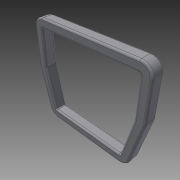
# Autodesk Inventor part: y_carryage_nut_holder_a_zip_tie
Saved by Autodesk Inventor 2014 (Build 180170000, 170)
## iProperties
Created: 2014-01-11
Part Number: y_carryage_nut_holder_a_zip_tie
Material: Generic
Document SubType Name: Modeling
Designer: buben
Density: 1 g/cm^3
Appearance: Default
Author: buben
Autodesk Inventor part; units mm, degrees
ref_plane "YZ Plane" through (0, 0, 0) normal (1, 0, 0) x (0, 1, 0)
ref_plane "XZ Plane" through (0, 0, 0) normal (0, 1, 0) x (-1, 0, 0)
ref_plane "XY Plane" through (0, 0, 0) normal (0, 0, 1) x (1, 0, 0)
sketch "Sketch1" plane through (0, 0, 0) normal (0, 1, 0) x (-1, 0, 0)
  line L0 (-7.8, 0) -> (7.8, 0)
  arc A0 (8, -0.2) -> (7.8, 0) centre (7.8, -0.2) ccw
  arc A1 (-7.8, 0) -> (-8, -0.2) centre (-7.8, -0.2) ccw
  line L1 (-8, -0.2) -> (-8, -6)
  line L2 (8, -0.2) -> (8, -6)
  arc A2 (-8, -6) -> (-7.9953, -6.043) centre (-7.8, -6) ccw
  arc A3 (7.9953, -6.043) -> (8, -6) centre (7.8, -6) ccw
  line L3 (-7.9953, -6.043) -> (-6.5, -12.843)
  line L4 (7.9953, -6.043) -> (6.5, -12.843)
  arc A4 (-6.5, -12.843) -> (-6.3047, -13) centre (-6.3047, -12.8) ccw
  line L5 (-6.3047, -13) -> (6.3047, -13)
  arc A5 (6.3047, -13) -> (6.5, -12.843) centre (6.3047, -12.8) ccw
  line L6 (-9.5, -6) -> (-9.5, -0.2)
  arc A6 (-7.8, 1.5) -> (-9.5, -0.2) centre (-7.8, -0.2) ccw
  line L7 (-7.8, 1.5) -> (7.8, 1.5)
  arc A7 (9.5, -0.2) -> (7.8, 1.5) centre (7.8, -0.2) ccw
  line L8 (9.5, -0.2) -> (9.5, -6)
  arc A8 (9.4603, -6.3651) -> (9.5, -6) centre (7.8, -6) ccw
  line L9 (9.4603, -6.3651) -> (7.965, -13.1651)
  arc A9 (6.3047, -14.5) -> (7.965, -13.1651) centre (6.3047, -12.8) ccw
  line L10 (6.3047, -14.5) -> (-6.3047, -14.5)
  arc A10 (-7.965, -13.1651) -> (-6.3047, -14.5) centre (-6.3047, -12.8) ccw
  line L11 (-7.965, -13.1651) -> (-9.4603, -6.3651)
  arc A11 (-9.5, -6) -> (-9.4603, -6.3651) centre (-7.8, -6) ccw
  point P0 (0, 0)
  point P1 (0, 0)
  point P2 (0, -13)
  dimension "d0" = 0.2
  dimension "d1" = 0.2
  dimension "d2" = 16
  dimension "d3" = 6
  dimension "d4" = 0.2
  dimension "d5" = 0.2
  dimension "d6" = 0.2
  dimension "d7" = 0.2
  dimension "d8" = 13
  dimension "d9" = 13
  dimension "d10" = 1.5
  constraints: 24 end point, 24 point on circle, 12 centre point, 12 tangent, 4 parallel, 2 midpoint, 2 perpendicular, 1 coincident, 1 horizontal, 1 horizontal alignment, 1 vertical alignment, 11 other
  measures "d0" radius of A1
  measures "d1" radius of A0
  measures "d2" distance of L2.start L1.start
  measures "d3" vertical distance of L1.end L0.start
  measures "d4" radius of A2
  measures "d5" radius of A4
  measures "d6" radius of A5
  measures "d7" radius of A3
  measures "d8" distance between parallel lines of L5 L0
  measures "d9" distance of L4.end L3.end
  measures "d10" distance between parallel lines of L1 L6
extrude "Extrusion1" add sketch "Sketch1" along normal blind 2
fillet "Fillet1" radius 0.3 48 edges at (9.0021, 2, 1.0021) (9.5, 2, -3.1) (9.4901, 2, -6.1836) (8.7127, 2, -9.7651) (7.3699, 2, -14.1249) (0, 2, -14.5) (-7.3699, 2, -14.1249) (-8.7127, 2, -9.7651) (-9.4901, 2, -6.1836) (-9.5, 2, -3.1) (-9.0021, 2, 1.0021) (0, 2, 1.5) (-7.9414, 2, -0.0586) (-8, 2, -3.1) (-7.9988, 2, -6.0216) (-7.2477, 2, -9.443) (-6.43, 2, -12.9559) (0, 2, -13) (6.43, 2, -12.9559) (7.2477, 2, -9.443) (7.9988, 2, -6.0216) (8, 2, -3.1) (7.9414, 2, -0.0586) (0, 2, 0) (-9.0021, 0, 1.0021) (-9.5, 0, -3.1) (-9.4901, 0, -6.1836) (-8.7127, 0, -9.7651) (-7.3699, 0, -14.1249) (0, 0, -14.5) (7.3699, 0, -14.1249) (8.7127, 0, -9.7651) (9.4901, 0, -6.1836) (9.5, 0, -3.1) (9.0021, 0, 1.0021) (0, 0, 1.5) (7.9414, 0, -0.0586) (8, 0, -3.1) (7.9988, 0, -6.0216) (7.2477, 0, -9.443) (6.43, 0, -12.9559) (0, 0, -13) (-6.43, 0, -12.9559) (-7.2477, 0, -9.443) (-7.9988, 0, -6.0216) (-8, 0, -3.1) (-7.9414, 0, -0.0586) (0, 0, 0)
equation "\"d1\" = d0"
equation "\"d4\" = d0"
equation "\"d5\" = d4"
equation "\"d6\" = d5"
equation "\"d7\" = d6"
body "Solid1"
